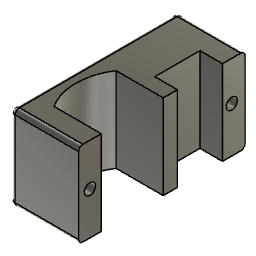
especial (Autodesk Fusion 360 design; units mm, degrees)
Autodesk Fusion 360 part; units mm, degrees
note: some values were not read from the file. Set by a fixed rule: which sketch regions a step uses.
sketch "Esboço1" plane through (0, 0, 0) normal (0, 0, 1) x (1, 0, 0)
  line L0 (-3.0001, 62) -> (21, 62)
  line L1 (21, 62) -> (21, 54)
  line L2 (21, 54) -> (13, 54)
  line L3 (13, 54) -> (13, 38)
  line L4 (13, 38) -> (21, 38)
  line L5 (21, 11) -> (21, 3)
  line L6 (-3, 3) -> (-3, 62)
  line L7 (-3, 3) -> (21, 3)
  line L8 (21, 33) -> (21, 38)
  line L9 (-3.0001, 62) -> (-3, 62)
  line L10 (21, 33) -> (1, 33)
  line L11 (1, 11) -> (21, 11)
  arc A0 (1, 22) -> (4.2967, 11) centre (21, 22) ccw
  arc A1 (4.2967, 33) -> (1, 22) centre (21, 22) ccw
  dimension "d2" = 16
  dimension "d3" = 8
  dimension "d5" = 8
  dimension "d8" = 8
  dimension "d10" = 8
  dimension "d35" = 5
  dimension "d36" = 24
  constraint perpendicular L1 L2
  constraint perpendicular L2 L3
  constraint perpendicular L3 L4
  constraint vertical L5
  constraint perpendicular L5 L7
  constraint perpendicular L8 L10
  constraint vertical L6
  constraint horizontal L10
  constraint coincident L11 A0.end
  constraint coincident L10 A1.start
  constraint coincident A0.centre A1.centre
  measures "d2" distance of L2.end L3.end
  measures "d3" distance of L1.end L2.end
  measures "d5" distance of L0.end L1.end
  measures "d8" distance of L4.end L3.end
  measures "d10" distance of L5.start L5.end
  measures "d35" distance of L4.end L8.start
  measures "d36" distance of L0.end L6.end
extrude "Extrusão1" add sketch "Esboço1" along normal blind 30
hole "Furo2" at (-3, 7, 15) direction (1, 0, 0) diameter 4 depth 25 tip angle 180
hole "Furo3" at (-3, 57.307, 16.094) direction (1, 0, 0) diameter 4 depth 25 tip angle 180
fillet "Arredondamento4" radius 1.5 8 edges at (9, 62, 30) (-3, 62, 15) (-3, 32.5, 30) (-3, 32.5, 0) (-3, 3, 15) (9, 3, 0) (9, 3, 30) (9, 62, 0)
